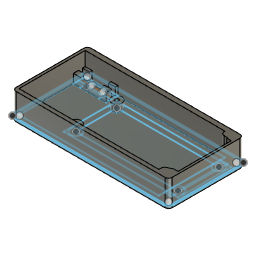
2_9inEpaperSmartDisplay (Autodesk Fusion 360 design; units mm, degrees)
Autodesk Fusion 360 part; units mm, degrees
sketch "Sketch1" plane through (0, 0, 0) normal (0, 0, 1) x (1, 0, 0)
  line L0 (2.8247, 48.5939) -> (87.8247, 48.5939)
  line L1 (89.8247, 46.5939) -> (89.8247, 7.8939)
  line L2 (87.8247, 5.8939) -> (2.8247, 5.8939)
  line L3 (0.8247, 7.8939) -> (0.8247, 46.5939)
  arc A0 (2.8247, 48.5939) -> (0.8247, 46.5939) centre (2.8247, 46.5939) ccw
  arc A1 (89.8247, 46.5939) -> (87.8247, 48.5939) centre (87.8247, 46.5939) ccw
  arc A2 (87.8247, 5.8939) -> (89.8247, 7.8939) centre (87.8247, 7.8939) ccw
  arc A3 (0.8247, 7.8939) -> (2.8247, 5.8939) centre (2.8247, 7.8939) ccw
  line L4 (2.2747, 45.8439) -> (82.0247, 45.8439)
  line L5 (82.0247, 45.8439) -> (82.0247, 8.0939)
  line L6 (82.0247, 8.0939) -> (2.2747, 8.0939)
  line L7 (2.2747, 8.0939) -> (2.2747, 45.8439)
  line L8 (82.0247, 43.3939) -> (86.0247, 43.3939)
  line L9 (86.0247, 43.3939) -> (86.0247, 11.3939)
  line L10 (86.0247, 11.3939) -> (82.0247, 11.3939)
  line L11 (82.0247, 11.3939) -> (82.0247, 43.3939)
  arc A4 (90.8247, 46.5939) -> (87.8247, 49.5939) centre (87.8247, 46.5939) ccw
  line L12 (2.8247, 49.5939) -> (87.8247, 49.5939)
  arc A5 (2.8247, 49.5939) -> (-0.1753, 46.5939) centre (2.8247, 46.5939) ccw
  line L13 (-0.1753, 7.8939) -> (-0.1753, 46.5939)
  arc A6 (-0.1753, 7.8939) -> (2.8247, 4.8939) centre (2.8247, 7.8939) ccw
  line L14 (87.8247, 4.8939) -> (2.8247, 4.8939)
  arc A7 (87.8247, 4.8939) -> (90.8247, 7.8939) centre (87.8247, 7.8939) ccw
  line L15 (90.8247, 46.5939) -> (90.8247, 7.8939)
  line L16 (23.3247, 42.8939) -> (88.5247, 42.8939)
  line L17 (88.5247, 42.8939) -> (88.5247, 12.5939)
  line L18 (88.5247, 12.5939) -> (23.3247, 12.5939)
  line L19 (23.3247, 12.5939) -> (23.3247, 42.8939)
  line L20 (85.0247, 16.0939) -> (26.8247, 16.0939)
  line L21 (26.8247, 16.0939) -> (26.8247, 39.3939)
  line L22 (26.8247, 39.3939) -> (85.0247, 39.3939)
  line L23 (85.0247, 39.3939) -> (85.0247, 16.0939)
  circle A8 centre (26.8247, 39.3939) radius 3
  circle A9 centre (26.8247, 39.3939) radius 1
  circle A10 centre (26.8247, 16.0939) radius 3
  circle A11 centre (26.8247, 16.0939) radius 1
  circle A12 centre (85.0247, 39.3939) radius 3
  circle A13 centre (85.0247, 39.3939) radius 1
  circle A14 centre (85.0247, 16.0939) radius 3
  circle A15 centre (85.0247, 16.0939) radius 1
  line L24 (2.2747, 45.8439) -> (21.0347, 45.8439)
  line L25 (21.0347, 45.8439) -> (21.0347, 40.6239)
  line L26 (21.0347, 40.6239) -> (2.2747, 40.6239)
  line L27 (2.2747, 40.6239) -> (2.2747, 45.8439)
  line L28 (11.6547, 40.6239) -> (11.6547, 45.8439) construction
  line L29 (21.0347, 43.2339) -> (2.2747, 43.2339) construction
  line L30 (11.6547, 43.2339) -> (16.1047, 43.2339) construction
  line L31 (16.1047, 43.2339) -> (16.1047, 41.4839) construction
  line L32 (14.8547, 41.4839) -> (11.6547, 41.4839) construction
  line L33 (11.6547, 41.4839) -> (11.6547, 43.2339) construction
  line L34 (16.1047, 41.4839) -> (8.4547, 41.4839)
  line L35 (7.2047, 42.7339) -> (7.2047, 43.7339)
  line L36 (8.4547, 44.9839) -> (14.8547, 44.9839)
  line L37 (16.1047, 43.7339) -> (16.1047, 42.7339)
  arc A16 (14.8547, 41.4839) -> (16.1047, 42.7339) centre (14.8547, 42.7339) ccw
  arc A17 (7.2047, 42.7339) -> (8.4547, 41.4839) centre (8.4547, 42.7339) ccw
  arc A18 (8.4547, 44.9839) -> (7.2047, 43.7339) centre (8.4547, 43.7339) ccw
  arc A19 (16.1047, 43.7339) -> (14.8547, 44.9839) centre (14.8547, 43.7339) ccw
  line L38 (21.0347, 44.3339) -> (2.2747, 44.3339)
  line L39 (21.0347, 42.1339) -> (2.2747, 42.1339)
  line L40 (21.0347, 44.3339) -> (17.0347, 44.3339)
  line L41 (17.0347, 44.3339) -> (17.0347, 45.8439)
  line L42 (17.0347, 45.8439) -> (21.0347, 45.8439)
  line L43 (21.0347, 45.8439) -> (21.0347, 44.3339)
  line L44 (21.0347, 42.1339) -> (17.0347, 42.1339)
  line L45 (17.0347, 42.1339) -> (17.0347, 39.1339)
  line L46 (17.0347, 39.1339) -> (21.0347, 39.1339)
  line L47 (21.0347, 39.1339) -> (21.0347, 42.1339)
  line L48 (2.2747, 42.1339) -> (6.2747, 42.1339)
  line L49 (6.2747, 42.1339) -> (6.2747, 39.1339)
  line L50 (6.2747, 39.1339) -> (2.2747, 39.1339)
  line L51 (2.2747, 39.1339) -> (2.2747, 42.1339)
  line L52 (2.2747, 44.3339) -> (6.2747, 44.3339)
  line L53 (6.2747, 44.3339) -> (6.2747, 45.8439)
  line L54 (6.2747, 45.8439) -> (2.2747, 45.8439)
  line L55 (2.2747, 45.8439) -> (2.2747, 44.3339)
  line L56 (6.2747, 39.1339) -> (17.0347, 39.1339)
  point P0 (0.8247, 48.5939)
  point P1 (89.8247, 48.5939)
  point P2 (0.8247, 5.8939)
  point P3 (7.2047, 41.4839)
  point P4 (16.1047, 44.9839)
  dimension "d1" = 89
  dimension "d2" = 42.7
  dimension "d3" = 2
  dimension "d4" = 2
  dimension "d5" = 2
  dimension "d6" = 79.75
  dimension "d7" = 37.75
  dimension "d8" = 81.2
  dimension "d9" = 40.5
  dimension "d10" = 4
  dimension "d11" = 32
  dimension "d12" = 5.5
  dimension "d17" = -1
  dimension "d22" = 65.2
  dimension "d23" = 30.3
  dimension "d24" = 66.5
  dimension "d25" = 37
  dimension "d26" = 3.5
  dimension "d27" = 6
  dimension "d28" = 2
  dimension "d29" = 6
  dimension "d30" = 2
  dimension "d31" = 6
  dimension "d32" = 2
  dimension "d33" = 6
  dimension "d34" = 2
  dimension "d50" = 18.76
  dimension "d51" = 5.22
  dimension "d52" = 4.45
  dimension "d53" = 1.75
  dimension "d54" = 8.9
  dimension "d55" = 3.5
  dimension "d56" = 1.25
  dimension "d57" = 1.1
  dimension "d58" = -1.1
  dimension "d61" = 4
  dimension "d62" = 4
  dimension "d63" = 3
  dimension "d64" = 4
  dimension "d65" = 3
  dimension "d66" = 4
  constraint horizontal L0
  constraint vertical L1
  constraint horizontal L2
  constraint vertical L3
  constraint coincident P0 L0
  constraint coincident P0 L3
  constraint tangent L0 A0
  constraint tangent L3 A0
  constraint coincident P1 L0
  constraint coincident P1 L1
  constraint tangent L0 A1
  constraint tangent L1 A1
  constraint equal A0 A1
  constraint tangent L1 A2
  constraint tangent L2 A2
  constraint coincident P2 L2
  constraint coincident P2 L3
  constraint tangent L2 A3
  constraint tangent L3 A3
  constraint horizontal L4
  constraint vertical L5
  constraint horizontal L6
  constraint vertical L7
  constraint horizontal L8
  constraint vertical L9
  constraint horizontal L10
  constraint vertical L11
  constraint coincident L5 L8.start
  constraint horizontal L16
  constraint vertical L17
  constraint horizontal L18
  constraint vertical L19
  constraint coincident L21.end L22.start
  constraint coincident L20.end L21.start
  constraint coincident L22.end L23.start
  constraint coincident L20.start L23.end
  constraint horizontal L24
  constraint vertical L25
  constraint horizontal L26
  constraint vertical L27
  constraint midpoint L26 L28.start
  constraint midpoint L24 L28.end
  constraint midpoint L25 L29.start
  constraint midpoint L27 L29.end
  constraint horizontal L30
  constraint vertical L31
  constraint horizontal L32
  constraint vertical L33
  constraint midpoint L29 L30.start
  constraint horizontal L34
  constraint vertical L35
  constraint horizontal L36
  constraint vertical L37
  constraint coincident L31.end L37
  constraint coincident L31.end L32
  constraint tangent L37 A16
  constraint tangent L32 A16
  constraint coincident P3 L34
  constraint coincident P3 L35
  constraint tangent L34 A17
  constraint tangent L35 A17
  constraint equal A16 A17
  constraint tangent L35 A18
  constraint tangent L36 A18
  constraint equal A16 A18
  constraint coincident P4 L36
  constraint coincident P4 L37
  constraint tangent L36 A19
  constraint tangent L37 A19
  constraint equal A16 A19
  constraint horizontal L40
  constraint vertical L41
  constraint horizontal L42
  constraint vertical L43
  constraint coincident L24 L41.end
  constraint horizontal L44
  constraint vertical L45
  constraint horizontal L46
  constraint vertical L47
  constraint horizontal L48
  constraint vertical L49
  constraint horizontal L50
  constraint vertical L51
  constraint horizontal L52
  constraint vertical L53
  constraint horizontal L54
  constraint vertical L55
  constraint coincident L24 L53.end
  constraint perpendicular L45 L56
  measures "d1" distance of P0 P1
  measures "d2" distance of P0 P2
  measures "d3" radius of A0
  measures "d4" radius of A2
  measures "d5" radius of A3
  measures "d6" distance of L4.start L4.end
  measures "d7" distance of L4.start L6.end
  measures "d8" distance of L3 L5
  measures "d9" distance of L0 L6
  measures "d10" distance of L8.start L8.end
  measures "d11" distance of L8.start L10.end
  measures "d12" distance of L2 L10
  measures "d22" distance of L16.start L16.end
  measures "d23" distance of L16.start L18.end
  measures "d24" distance of L1 L19
  measures "d25" distance of L2 L16
  measures "d27" diameter of A8
  measures "d28" diameter of A9
  measures "d29" diameter of A10
  measures "d30" diameter of A11
  measures "d31" diameter of A12
  measures "d32" diameter of A13
  measures "d33" diameter of A14
  measures "d34" diameter of A15
  measures "d50" distance of L4.start L24.end
  measures "d51" distance of L4.start L26.end
  measures "d52" distance of L30.start L30.end
  measures "d53" distance of L30.start L32.end
  measures "d54" distance of L31.end P3
  measures "d55" distance of L31.end P4
  measures "d56" radius of A16
  measures "d61" distance of L38.start L40.end
  measures "d62" distance of L39.start L44.end
  measures "d63" distance of L39.start L46.end
  measures "d64" distance of L39.end L48.end
  measures "d65" distance of L39.end L50.end
  measures "d66" distance of L38.end L52.end
extrude "Extrude1" add sketch "Sketch1" along normal blind 13 contours L0 L1 L2 L3 A0 A1 A2 A3
extrude "Extrude2" add sketch "Sketch1" against normal blind 2 contours L0 L1 L2 L3 A0 A1 A2 A3 | L4 L7 L24 L27 L38 L52 L53 L54 L55 | L4 L24 L36 A18 A19 L38 L41 L53 | L7 L27 L35 A17 A18 L38 L39 L48 L52 | L4 L24 L25 L38 L40 L41 L42 L43 | L7 L26 L27 L39 L48 L49 L51 | L4 L5 L6 L7 L11 L16 L18 L19 L25 L43 L46 L47 L50 L56 | L25 L37 A16 A19 L38 L39 L40 L44 | L35 L37 A16 A17 A18 A19 L38 L39 | L36 A18 A19 L38 | L7 L26 L49 L50 L51 | L26 L34 A16 A17 L39 L45 L49 | L26 L45 L49 L56 | L34 A16 A17 L39 | L5 L8 L9 L11 L16 | L25 L26 L39 L44 L45 L47 | L26 L45 L46 L47 | L5 L9 L11 L16 A12 | L5 L11 L16 L18 L19 L20 L21 L22 A8 A10 | L5 L11 L23 A12 A14 | L5 L11 L20 L21 L22 A8 A10 | L9 L22 A12 A13 | L22 L23 A12 A13 | L9 L16 L17 L18 A12 A14 | L5 L9 L10 L11 L18 | L5 L9 L11 L18 A14 | L20 L23 A14 A15 | L9 L20 A14 A15 | L21 L22 A8 A9 | L21 L22 A8 A9 | L22 L23 A13 | L22 L23 A13 | L9 A12 | L9 L23 A12 A14 | L9 L23 A12 A13 | L20 L23 A15 | L20 L23 A15 | L20 L21 A10 A11 | L20 L21 A10 A11 | L9 L23 A14 A15 | L9 A14 | L21 L22 A9 | L21 L22 A9 | L20 L21 A11 | L20 L21 A11
extrude "Extrude4" add sketch "Sketch1" along normal blind 4 contours L9 L22 A12 A13 | L22 L23 A12 A13 | L20 L23 A14 A15 | L9 L20 A14 A15 | L21 L22 A8 A9 | L21 L22 A8 A9 | L9 A12 | L9 L23 A12 A13 | L20 L21 A10 A11 | L20 L21 A10 A11 | L9 L23 A14 A15 | L9 A14
extrude "Extrude5" [suppressed]
fillet "Fillet1" radius 2 1 edges at (82.0247, 43.3939, 6.5)
fillet "Fillet2" radius 2 1 edges at (82.0247, 11.3939, 6.5)
extrude "Extrude6" cut sketch "Sketch1" along normal blind 26 from surface at 4 contours L5 L9 L11 L16 A12 | L5 L11 L23 A12 A14 | L9 L22 A12 A13 | L22 L23 A12 A13 | L9 L16 L17 L18 A12 A14 | L5 L9 L11 L18 A14 | L20 L23 A14 A15 | L9 L20 A14 A15 | L22 L23 A13 | L22 L23 A13 | L9 A12 | L9 L23 A12 A14 | L9 L23 A12 A13 | L20 L23 A15 | L20 L23 A15 | L9 L23 A14 A15 | L9 A14
extrude "Extrude7" cut sketch "Sketch1" along normal blind 13 contours L22 L23 A13 | L22 L23 A13 | L20 L23 A15 | L20 L23 A15
chamfer "Chamfer2" [suppressed]
extrude "Extrude8" cut sketch "Sketch1" against normal blind 9 contours L35 L37 A16 A17 A18 A19 L38 L39 | L36 A18 A19 L38 | L34 A16 A17 L39
extrude "Extrude9" add sketch "Sketch1" along normal blind 5 contours L4 L7 L24 L27 L38 L52 L53 L54 L55 | L4 L24 L25 L38 L40 L41 L42 L43 | L7 L26 L27 L39 L48 L49 L51 | L7 L26 L49 L50 L51 | L26 L45 L49 L56 | L25 L26 L39 L44 L45 L47 | L26 L45 L46 L47
fillet "Fillet3" [no effect]
fillet "Fillet4" radius 34.5 1 edges at (86.0247, 11.3939, 6.5)
fillet "Fillet7" [no effect]
fillet "Fillet8" [no effect]
fillet "Fillet9" [no effect]
equation "d13 = BoxHeight"
equation "d35 = BoxHeight - ComponentHeight"
equation "d44 = BoxHeight - 9 mm"
equation "d45 = BoxHeight * 2"
equation "d47 = BoxHeight"
equation "BoxHeight = 13 mm" comment "The total inside height of the box"
equation "ComponentHeight = 9 mm" comment "The height from the underside of the glass to the bottom of the raspberry board at screwholes"
